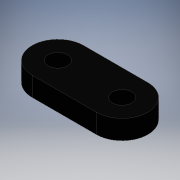
# Autodesk Inventor part: Updown_link
Saved by Autodesk Inventor 2016 (Build 200138000, 138)
## iProperties
Created: 2015-12-07
Part Number: Updown_link
Material: Generic
Document SubType Name: Modeling
Designer: lk8187
Density: 1 g/cm^3
Appearance: Smooth - Black(1)
Author: lk8187
Autodesk Inventor part; units mm, degrees
ref_plane "YZ Plane" through (0, 0, 0) normal (1, 0, 0) x (0, 1, 0)
ref_plane "XZ Plane" through (0, 0, 0) normal (0, 1, 0) x (-1, 0, 0)
ref_plane "XY Plane" through (0, 0, 0) normal (0, 0, 1) x (1, 0, 0)
sketch "Sketch1" plane through (0, 0, 0) normal (0, 0, 1) x (1, 0, 0)
  line L0 (0, 0) -> (10, 0) construction
  line L1 (0, -4) -> (10, -4)
  line L2 (10, 4) -> (0, 4)
  arc A0 (0, 4) -> (0, -4) centre (0, 0) ccw
  arc A1 (10, -4) -> (10, 4) centre (10, 0) ccw
  point P0 (5, 0)
  dimension "d0" = 10
  dimension "d1" = 4
  constraints: 8 end point, 4 point on circle, 4 tangent, 2 centre point, 2 coincident, 1 horizontal, 1 midpoint, 1 parallel
  measures "d0" distance of L0.start L0.end
  measures "d1" radius of A0
extrude "Extrusion1" add sketch "Sketch1" against normal blind 3
hole "Hole1" at (0, 0, 0) at (10, 0, 0) direction (0, 0, -1) diameter 3 depth 8 tip angle 118
body "Solid1"
